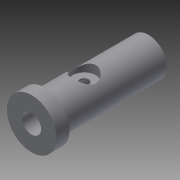
# Autodesk Inventor part: dc_to_omni_coupler
Saved by Autodesk Inventor 2015 (Build 190159000, 159)
## iProperties
Created: 2017-09-27
Part Number: dc_to_omni_coupler
Material: Generic
Document SubType Name: Modeling
Designer: Anshul
Density: 1 g/cm^3
Appearance: Default
Author: Anshul
Autodesk Inventor part; units mm, degrees
ref_plane "YZ Plane" through (0, 0, 0) normal (1, 0, 0) x (0, 1, 0)
ref_plane "XZ Plane" through (0, 0, 0) normal (0, 1, 0) x (-1, 0, 0)
sketch "Sketch1" plane through (0, 0, 0) normal (0, 1, 0) x (-1, 0, 0)
  line L0 (0, -40) -> (0, 0)
  line L1 (0, 0) -> (0, -18)
  circle A0 centre (0, -18) radius 1.55
  line L2 (0, -18) -> (0, -26.5)
  line L3 (0, -40) -> (0, -32)
  line L4 (0, -32) -> (1.5, -32)
  line L5 (1.5, -32) -> (1.5, -40)
  line L6 (0, 0) -> (6.4, 0)
  line L7 (6.4, 0) -> (6.4, -40)
  line L8 (6.4, -40) -> (1.5, -40)
  line L9 (6.4, -40) -> (7.9, -40)
  line L10 (7.9, -40) -> (7.9, 0)
  line L11 (7.9, 0) -> (6.4, 0)
  line L12 (6.4, 0) -> (4.9, 0)
  line L13 (4.9, 0) -> (4.9, -40)
  line L14 (4.9, -40) -> (6.4, -40)
  line L15 (0, 0) -> (3.15, 0)
  line L16 (3.15, 0) -> (3.15, -26.5)
  line L17 (3.15, -26.5) -> (0, -26.5)
  line L18 (7.9, 0) -> (7.9, -20)
  line L19 (7.9, -20) -> (6.4, -20)
  line L20 (6.4, -20) -> (4.9, -20)
  dimension "d3" = 18
  dimension "d4" = 3.1
  dimension "d5" = 8.5
  dimension "d6" = 8
  dimension "d7" = 1.5
  dimension "d22" = 6.4
  dimension "d27" = 1.5
  dimension "d28" = 1.5
  dimension "d35" = 3.15
  dimension "d45" = 20
  constraints: 42 end point, 9 perpendicular, 6 point on line, 3 midpoint, 2 horizontal, 1 centre point, 1 coincident
  measures "d3" distance of L0.end L1.end
  measures "d4" diameter of A0
  measures "d5" distance of L2.start L2.end
  measures "d6" distance of L0.start L3.end
  measures "d7" distance of L3.end L4.end
  measures "d22" distance of L0.end L6.end
  measures "d27" distance of L7.end L9.end
  measures "d28" distance of L6.end L12.end
  measures "d35" distance of L0.end L15.end
  measures "d45" distance of L10.end L18.end
revolve "Revolution3" add sketch "Sketch1" angle 360 about axis through (0, 0, 0) along (0, 0, -1) contours L0 L17 L16 L6 L13 L8 L5 L4 | L13 L20 L7 L8 | L6 L7 L20 L13
extrude "Extrusion8" cut sketch "Sketch1" along normal mid plane 15 contours A0 L0 | L0 A0
ref_plane "Work Plane3" through (0, 6.4, -20) normal (0, 1, 0) x (-1, 0, 0)
sketch "Sketch4" plane through (0, 6.4, -20) normal (0, 1, 0) x (-1, 0, 0)
  line L0 (0, 20) -> (0, 2)
  circle A0 centre (0, 2) radius 4
  dimension "d41" = 18
  dimension "d42" = 8
  constraints: 2 end point, 1 centre point, 1 coincident, 1 vertical
  measures "d41" distance of L0.start L0.end
  measures "d42" diameter of A0
extrude "Extrusion9" cut sketch "Sketch4" against normal blind 3
extrude "Extrusion10" add sketch "Sketch1" along normal mid plane 3 contours L6 L7 L20 L13 | L11 L10 L19 L7
sketch "Sketch5" plane through (-7.9, 1.5, 0) normal (0, 0, 1) x (1, 0, 0)
  circle A0 centre (7.9, -1.5) radius 3.25
  circle A1 centre (7.9, -1.5) radius 1.5 projected
  circle A2 centre (7.9, -1.5) radius 8.5
  dimension "d48" = 6.5
  dimension "d51" = 17
  constraints: 2 centre point, 2 coincident
  measures "d48" diameter of A0
  measures "d51" diameter of A2
extrude "Extrusion11" cut sketch "Sketch5" against normal blind 26.5 contours A0 | A1
extrude "Extrusion12" add sketch "Sketch5" against normal blind 4.5 contours A2
body "Solid3"
